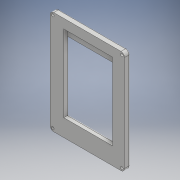
# Autodesk Inventor part: LidTest02
Saved by Autodesk Inventor 2018.3 (Build 223285000, 285)
## iProperties
Created: 2022-01-12
Part Number: LidTest02
Material: Generic
Document SubType Name: Modeling
Designer: Stewart Alexander
Density: 1 g/cm^3
Appearance: Default
Author: Stewart Alexander
Autodesk Inventor part; units mm, degrees
ref_plane "YZ Plane" through (0, 0, 0) normal (1, 0, 0) x (0, 1, 0)
ref_plane "XZ Plane" through (0, 0, 0) normal (0, 1, 0) x (-1, 0, 0)
ref_plane "XY Plane" through (0, 0, 0) normal (0, 0, 1) x (1, 0, 0)
sketch "Sketch1" plane through (0, 0, 0) normal (0, 1, 0) x (-1, 0, 0)
  line L0 (0, 0) -> (83.3, 0)
  line L1 (83.3, 0) -> (83.3, -115.6)
  line L2 (83.3, -115.6) -> (0, -115.6)
  line L3 (0, -115.6) -> (0, 0)
  dimension "d0" = 115.6
  dimension "d1" = 83.3
  constraints: 8 end point, 2 parallel, 1 horizontal, 1 perpendicular
  measures "d0" distance of L0.end L1.end
  measures "d1" distance of L1.end L2.end
extrude "Lid Body" add sketch "Sketch1" along normal blind 6
fillet "4mm Fillet" radius 4 4 edges at (0, 3, -115.6) (-83.3, 3, -115.6) (-83.3, 3, 0) (0, 3, 0)
sketch "Sketch2" plane through (0, 6, 0) normal (0, 1, 0) x (1, 0, 0)
  circle A0 centre (-80.3, 3) radius 1.5
  line L0 (-83.3, 115.6) -> (-83.3, 0) projected
  line L1 (-83.3, 0) -> (0, 0) projected
  line L2 (-83.3, 57.8) -> (0, 57.8)
  line L3 (0, 0) -> (0, 115.6) projected
  line L4 (-41.65, 0) -> (-41.65, 124)
  circle A1 centre (-80.3, 112.6) radius 1.5
  circle A2 centre (-3, 3) radius 1.5
  circle A3 centre (-3, 112.6) radius 1.5
  dimension "d5" = 3
  dimension "d6" = 3
  dimension "d7" = 3
  constraints: 4 centre point, 4 end point, 3 midpoint, 3 symmetric about line, 1 vertical, 3 other
  measures "d5" diameter of A0
  measures "d6" distance from line of L0 A0.centre
  measures "d7" distance from line of L1 A0.centre
extrude "3mm Mounting Holes" cut sketch "Sketch2" against normal through all contours A0 | A1 | A2 | A3
sketch "Sketch3" plane through (0, 6, 0) normal (0, 1, 0) x (1, 0, 0)
  line L0 (-83.3, 0) -> (0, 0) projected
  line L1 (0, 0) -> (0, 115.6) projected
  line L2 (0, 115.6) -> (-83.3, 115.6) projected
  line L3 (-83.3, 115.6) -> (-83.3, 0) projected
  line L4 (-78.3, 5) -> (-5, 5)
  line L5 (-5, 5) -> (-5, 110.6)
  line L6 (-5, 110.6) -> (-78.3, 110.6)
  line L7 (-78.3, 110.6) -> (-78.3, 5)
  line L8 (-68, 19.3) -> (-13.5, 19.3)
  line L9 (-13.5, 19.3) -> (-13.5, 96.3)
  line L10 (-13.5, 96.3) -> (-68, 96.3)
  line L11 (-68, 96.3) -> (-68, 19.3)
  dimension "d11" = 5
  dimension "d12" = 54.5
  dimension "d13" = 77
  dimension "d14" = 10.3
  dimension "d18" = 14.3
  constraints: 16 end point, 2 parallel, 1 horizontal, 1 perpendicular, 3 other
  measures "d11" distance between parallel lines of L3 L7
  measures "d12" distance of L9.end L10.end
  measures "d13" distance of L8.end L9.end
  measures "d14" distance between parallel lines of L7 L11
  measures "d18" distance between parallel lines of L6 L10
extrude "Screen Cut-Out" cut sketch "Sketch3" against normal through all contours L11 L10 L9 L8
fillet "Fillet3" radius 1 8 edges at (-82.1284, 6, -1.1716) (-41.65, 6, 0) (-1.1716, 6, -1.1716) (0, 6, -57.8) (-1.1716, 6, -114.4284) (-41.65, 6, -115.6) (-82.1284, 6, -114.4284) (-83.3, 6, -57.8)
fillet "Fillet4" radius 2 4 edges at (-40.75, 6, -19.3) (-68, 6, -57.8) (-40.75, 6, -96.3) (-13.5, 6, -57.8)
sketch "Sketch4" plane through (0, 0, 0) normal (0, -1, 0) x (1, 0, 0)
  line L0 (-68, -19.3) -> (-13.5, -19.3) projected
  line L1 (-13.5, -19.3) -> (-68, -19.3)
  line L2 (-68, -19.3) -> (-68, -10.3)
  line L3 (-68, -10.3) -> (-13.5, -10.3)
  line L4 (-13.5, -10.3) -> (-13.5, -19.3)
  point P0 (0, 0)
  dimension "d21" = 9
  constraints: 8 end point, 2 parallel, 1 horizontal, 1 perpendicular
  measures "d21" distance of L1.end L2.end
extrude "Extrusion4" cut sketch "Sketch4" against normal blind 4
body "Solid1"
